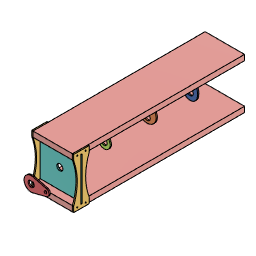
awesomeAutomataCAD (Autodesk Fusion 360 design; units mm, degrees)
Autodesk Fusion 360 part; units mm, degrees
note: some values were not read from the file. Set by a fixed rule: which sketch regions a step uses.
sketch "Sketch1" plane through (0, 0, 0) normal (0, 1, 0) x (1, 0, 0) in component "board"
  line L0 (0, -19.304) -> (139.7, -19.304)
  line L1 (139.7, -19.304) -> (139.7, 0)
  line L2 (139.7, 0) -> (0, 0)
  line L3 (0, 0) -> (0, -19.304)
  dimension "d5" = 139.7
  dimension "d6" = 19.304
  constraint horizontal L0
  constraint vertical L1
  constraint horizontal L2
  constraint vertical L3
  constraint coincident L2.end L3.start
  measures "d5" distance of L0.start L0.end
  measures "d6" distance of L0.start L2.end
extrude "Extrude1" add sketch "Sketch1" along normal blind 609.6 makes body 1 in component "board"
sketch "Sketch2" plane through (139.7, 0, 0) normal (1, 0, 0) x (0, 1, 0) in component "board"
  line L0 (0, 19.304) -> (0, 0)
  line L1 (0, 0) -> (609.6, 0)
  line L2 (609.6, 0) -> (609.6, 19.304)
  line L3 (609.6, 19.304) -> (0, 19.304)
  line L4 (25.4, 19.304) -> (25.4, 12.954)
  line L5 (25.4, 12.954) -> (29.8, 12.954)
  line L6 (29.8, 12.954) -> (29.8, 19.304)
  dimension "d9" = 4.4
  dimension "d10" = 6.35
  dimension "d11" = 25.4
  constraint coincident L3 L4.start
  constraint perpendicular L3 L4
  constraint perpendicular L4 L5
  constraint coincident L3 L6.end
  constraint perpendicular L3 L6
  measures "d9" distance of L4.end L5.end
  measures "d10" distance of L5.end L6.end
  measures "d11" distance of L0.start L4.start
extrude "Extrude2" cut sketch "Sketch2" against normal through all contours L3 L4 L5 L6 bodies 1 in component "board"
copy_body "CopyPasteBodies1" bodies 1 makes body 2 in component "board"
move_body "Move1" bodies 2 to x (1, 0, 0) y (0, -1, 0) z (0, 0, -1) at (0, 0, 0) in component "board"
move_body "Move2" bodies 2 to x (-1, 0, 0) y (0, -1, 0) z (0, 0, 1) at (0, 0, 0) in component "board"
move_body "Move3" bodies 2 to x (1, 0, 0) y (0, 1, 0) z (0, 0, 1) at (139.7, 0, 38.608) in component "board"
move_body "Move4" bodies 2 to x (1, 0, 0) y (0, 1, 0) z (0, 0, 1) at (0, 0, 139.7) in component "board"
sketch "Sketch1 (2)" plane through (0, 0, 0) normal (1, 0, 0) x (0, 1, 0) in component "sideSupport"
  line L0 (29.8, 165.354) -> (29.8, 159.004)
  line L1 (29.8, 159.004) -> (609.6, 159.004)
  line L2 (609.6, 159.004) -> (609.6, 178.308)
  line L3 (609.6, 178.308) -> (0, 178.308)
  line L4 (0, 178.308) -> (0, 159.004)
  line L5 (0, 159.004) -> (25.4, 159.004)
  line L6 (25.4, 159.004) -> (25.4, 165.354)
  line L7 (25.4, 165.354) -> (29.8, 165.354)
  line L8 (29.8, 19.304) -> (29.8, 12.954)
  line L9 (29.8, 12.954) -> (25.4, 12.954)
  line L10 (25.4, 12.954) -> (25.4, 19.304)
  line L11 (25.4, 19.304) -> (0, 19.304)
  line L12 (0, 19.304) -> (0, 0)
  line L13 (0, 0) -> (609.6, 0)
  line L14 (609.6, 0) -> (609.6, 19.304)
  line L15 (609.6, 19.304) -> (29.8, 19.304)
  line L16 (0, 159.004) -> (0, 178.308)
  line L17 (0, 178.308) -> (55.2, 178.308)
  line L18 (55.2, 178.308) -> (55.2, 159.004)
  line L19 (0, 0) -> (55.2, 0)
  line L20 (55.2, 0) -> (55.2, 19.304)
  circle A0 centre (12.7, 168.656) radius 2.032
  circle A1 centre (42.5, 168.656) radius 2.032
  circle A2 centre (12.7, 9.652) radius 2.032
  circle A3 centre (42.5, 9.652) radius 2.032
  line L21 (12.7, 159.004) -> (12.7, 19.304) construction
  line L22 (42.5, 19.304) -> (42.5, 159.004) construction
  spline S0 degree 5 poles (55.2, 19.304) (54.2367, 22.098) (52.3943, 27.686) (49.8831, 36.068) (47.0478, 47.244) (44.4169, 61.214) (42.7808, 75.184) (42.2207, 89.154) (42.7808, 103.124) (44.4169, 117.094) (47.0478, 131.064) (49.8831, 142.24) (52.3943, 150.622) (54.2367, 156.21) (55.2, 159.004) knots 0 0 0 0 0 0 0.1 0.2 0.3 0.4 0.5 0.6 0.7 0.8 0.9 1 1 1 1 1 1
  spline S1 degree 5 poles (0, 159.004) (0.9633, 156.21) (2.8057, 150.622) (5.3169, 142.24) (8.1522, 131.064) (10.7831, 117.094) (12.4192, 103.124) (12.9793, 89.154) (12.4192, 75.184) (10.7831, 61.214) (8.1522, 47.244) (5.3169, 36.068) (2.8057, 27.686) (0.9633, 22.098) (0, 19.304) knots 0 0 0 0 0 0 0.1 0.2 0.3 0.4 0.5 0.6 0.7 0.8 0.9 1 1 1 1 1 1
  line L23 (29.8, 159.004) -> (29.8, 19.304)
  line L24 (25.4, 19.304) -> (25.4, 159.004)
  point P0 (42.5, 89.154)
  point P1 (12.7, 89.154)
  dimension "d18" = 55.2
  dimension "d19" = 55.2
  dimension "d20" = 4.064
  dimension "d21" = 9.652
  dimension "d22" = 12.7
  dimension "d23" = 4.064
  dimension "d24" = 9.652
  dimension "d25" = 12.7
  dimension "d26" = 4.064
  dimension "d27" = 4.064
  dimension "d28" = 9.652
  dimension "d29" = 9.652
  dimension "d30" = 12.7
  dimension "d31" = 12.7
  dimension "d32" = 12.7
  constraint coincident L4.end L5.start
  constraint coincident L3.end L4.start
  constraint perpendicular L16 L17
  constraint coincident L1 L18.end
  constraint perpendicular L1 L18
  constraint coincident L12.end L13.start
  constraint perpendicular L12 L19
  constraint coincident L15 L20.end
  constraint perpendicular L15 L20
  constraint midpoint L5 L21.start
  constraint midpoint L11 L21.end
  constraint coincident L15 L22.start
  constraint coincident L1 L22.end
  constraint perpendicular L1 L22
  constraint midpoint L22 P0
  constraint midpoint L21 P1
  constraint coincident L11.end L12.start
  constraint coincident L0.end L1.start
  constraint coincident L8.start L15.end
  constraint coincident L10.end L11.start
  constraint coincident L5.end L6.start
  measures "d18" distance of L3.end L17.end
  measures "d19" distance of L12.end L19.end
  measures "d20" diameter of A0
  measures "d21" distance of L17 A0.centre
  measures "d22" distance of L16 A0.centre
  measures "d23" diameter of A1
  measures "d24" distance of L17 A1.centre
  measures "d25" distance of L18 A1.centre
  measures "d26" diameter of A2
  measures "d27" diameter of A3
  measures "d28" distance of L11 A2.centre
  measures "d29" distance of L15 A3.centre
  measures "d30" distance of L12 A2.centre
  measures "d31" distance of L20 A3.centre
  measures "d32" distance of L18.end L22
extrude "Extrude1'" add sketch "Sketch1 (2)" against normal blind 4.4 separate body contours L0 L1 L3 L4 L5 L6 L7 L16 L17 L18 | L1 L15 S0 L23 | L8 L9 L10 L11 L12 L13 L15 L19 L20 | L5 L11 S1 L24 makes body 3 in component "sideSupport"
copy_body "CopyPasteBodies1'" bodies 3 makes body 4 in component "sideSupport"
move_body "Move1'" bodies 4 to x (1, 0, 0) y (0, 1, 0) z (0, 0, 1) at (144.1, 0, 0) in component "sideSupport"
sketch "Sketch2 (2)" plane through (0, 29.8, 0) normal (0, -1, 0) x (1, 0, 0) in component "midSupport"
  line L0 (0, 12.954) -> (0, 165.354)
  line L1 (0, 165.354) -> (-4.4, 165.354)
  line L2 (-4.4, 165.354) -> (-4.4, 12.954)
  line L3 (-4.4, 12.954) -> (0, 12.954)
  line L4 (144.1, 12.954) -> (144.1, 165.354)
  line L5 (144.1, 165.354) -> (139.7, 165.354)
  line L6 (139.7, 165.354) -> (139.7, 12.954)
  line L7 (139.7, 12.954) -> (144.1, 12.954)
  line L8 (139.7, 159.004) -> (139.7, 165.354)
  line L9 (139.7, 165.354) -> (0, 165.354)
  line L10 (0, 165.354) -> (0, 159.004)
  line L11 (0, 159.004) -> (139.7, 159.004)
  line L12 (0, 19.304) -> (0, 12.954)
  line L13 (0, 12.954) -> (139.7, 12.954)
  line L14 (139.7, 12.954) -> (139.7, 19.304)
  line L15 (139.7, 19.304) -> (0, 19.304)
  line L16 (144.1, 12.954) -> (-4.4, 165.354) construction
  line L17 (-4.4, 12.954) -> (144.1, 165.354) construction
  circle A0 centre (69.85, 89.154) radius 10.795
  dimension "d35" = 21.59
  constraint coincident L4.start L7.end
  constraint coincident L1.end L2.start
  constraint coincident L2.end L3.start
  constraint coincident L4.end L5.start
  constraint midpoint L17 A0.centre
  measures "d35" diameter of A0
extrude "Extrude1''" add sketch "Sketch2 (2)" along normal blind 4.4 separate body makes body 5 in component "midSupport"
ref_plane "WorkPlane1" through (69.85, 182.2, 89.154) normal (0, 1, 0) x (-1, 0, 0) in component "pearCam"
sketch "Sketch1 (3)" plane through (69.85, 182.2, 95.504) normal (0, 1, 0) x (1, 0, 0) in component "pearCam"
  circle A0 centre (0, 6.35) radius 10.795
  line L0 (74.25, 82.55) -> (-74.25, 82.55)
  line L1 (-74.25, 82.55) -> (-74.25, -69.85)
  line L2 (-74.25, -69.85) -> (74.25, -69.85)
  line L3 (74.25, -69.85) -> (74.25, 82.55)
  circle A1 centre (0, 6.35) radius 21.59
  circle A2 centre (0, -31.75) radius 6.35
  line L4 (19.7876, -2.286) -> (5.8199, -34.29)
  line L5 (-19.7876, -2.286) -> (-5.8199, -34.29)
  line L6 (0, -31.75) -> (0, 6.35) construction
  dimension "d40" = 43.18
  dimension "d41" = 12.7
  dimension "d42" = 38.1
  constraint concentric A0 A1
  constraint coincident A1 L4.start
  constraint coincident A2 L4.end
  constraint tangent A2 L4
  constraint coincident A1 L5.start
  constraint coincident A2 L5.end
  constraint tangent A2 L5
  constraint coincident A2.centre L6.start
  constraint coincident A0.centre A1.centre
  constraint vertical L6
  constraint tangent A1 L5
  constraint tangent A1 L4
  measures "d40" diameter of A1
  measures "d41" diameter of A2
  measures "d42" distance of A0.centre A2.centre
extrude "Extrude1'''" add sketch "Sketch1 (3)" along normal blind 4.4 separate body contours A1 | A1 A2 L4 L5 | A2 makes body 6 in component "pearCam"
ref_plane "WorkPlane1" through (69.85, 334.6, 89.154) normal (0, 1, 0) x (-1, 0, 0) in component "eccentricCam"
sketch "Sketch1 (4)" plane through (69.85, 334.6, 89.154) normal (0, 1, 0) x (1, 0, 0) in component "eccentricCam"
  circle A0 centre (0, 0) radius 10.795
  circle A1 centre (0, -12.7) radius 31.75
  line L0 (0, 0) -> (0, -21.8372) construction
  dimension "d46" = 63.5
  dimension "d47" = 12.7
  constraint coincident A0.centre L0.start
  constraint vertical L0
  constraint coincident A1.centre L0
  measures "d46" diameter of A1
  measures "d47" distance of A0.centre A1.centre
extrude "Extrude1''''" add sketch "Sketch1 (4)" along normal blind 4.4 separate body makes body 7 in component "eccentricCam"
ref_plane "WorkPlane1" through (69.85, 487, 89.154) normal (0, 1, 0) x (-1, 0, 0) in component "snailCam"
sketch "Sketch1 (5)" plane through (69.85, 487, 89.154) normal (0, 1, 0) x (1, 0, 0) in component "snailCam"
  circle A0 centre (0, 0) radius 10.795
  circle A1 centre (0, 0) radius 25.4
  line L0 (0, 0) -> (0, -42.5762)
  arc A2 (7.1494, -46.0115) -> (24.5934, 6.35) centre (-24.5934, -6.35) ccw
  arc A3 (0, -42.5762) -> (7.1494, -46.0115) centre (4.4, -42.5762) ccw
  point P0 (0, -50.8)
  dimension "d51" = 50.8
  dimension "d52" = 50.8
  dimension "d53" = 50.8
  dimension "d54" = 4.4
  constraint concentric A0 A1
  constraint coincident A0.centre A1.centre
  constraint vertical L0
  constraint coincident A1 A2.end
  constraint tangent A1 A2
  constraint coincident P0 L0
  constraint coincident P0 A2
  constraint tangent L0 A3
  constraint tangent A2 A3
  measures "d51" diameter of A1
  measures "d52" distance of A0.centre P0
  measures "d53" radius of A2
  measures "d54" radius of A3
extrude "Extrude1'''''" add sketch "Sketch1 (5)" along normal blind 4.4 separate body makes body 8 in component "snailCam"
ref_plane "WorkPlane1" through (0, -76.2, 0) normal (0, 1, 0) x (0, 0, 1) in component "handle"
sketch "Sketch1 (6)" plane through (0, -76.2, 0) normal (0, 1, 0) x (1, 0, 0) in component "handle"
  circle A0 centre (69.85, -89.154) radius 10.795
  circle A1 centre (69.85, -89.154) radius 25.4
  line L0 (69.85, -89.154) -> (120.65, -89.154) construction
  circle A2 centre (120.65, -89.154) radius 12.7
  circle A3 centre (120.65, -89.154) radius 4.7625
  line L1 (76.2, -64.5606) -> (123.825, -76.8573)
  line L2 (123.825, -101.4507) -> (76.2, -113.7474)
  line L3 (45.8289, -97.409) -> (93.8711, -97.409)
  dimension "d58" = 50.8
  dimension "d59" = 50.8
  dimension "d60" = 25.4
  dimension "d61" = 9.525
  dimension "d62" = 8.255
  constraint concentric A0 A1
  constraint coincident A0.centre A1.centre
  constraint horizontal L0
  constraint coincident L0.end A2.centre
  constraint concentric A2 A3
  constraint coincident A1 L1.start
  constraint coincident A2 L1.end
  constraint coincident A2 L2.start
  constraint coincident A1 L2.end
  constraint tangent A1 L1
  constraint tangent A2 L1
  constraint tangent A2 L2
  constraint tangent A1 L2
  constraint coincident A1 L3.start
  constraint coincident A1 L3.end
  constraint horizontal L3
  measures "d58" diameter of A1
  measures "d59" distance of A0.centre L0.end
  measures "d60" diameter of A2
  measures "d61" diameter of A3
  measures "d62" distance of A0.centre L3
extrude "Extrude1''''''" add sketch "Sketch1 (6)" along normal blind 4.4 separate body contours A0 A1 L3 | A0 L3 | A0 A1 L3 | A1 A2 L1 L2 | A2 picked at (71.7619, -97.7057) makes body 9 in component "handle"
sketch "Sketch1 (7)" plane through (0, -76.2, 0) normal (0, -1, 0) x (1, 0, 0) in component "projectedFront"
  arc A0 (62.8939, 97.409) -> (76.8061, 97.409) centre (69.85, 89.154) ccw
  line L0 (62.8939, 97.409) -> (76.8061, 97.409)
  circle A1 centre (120.65, 89.154) radius 4.7625
  arc A2 (76.2, 113.7474) -> (76.2, 64.5606) centre (69.85, 89.154) ccw
  line L1 (76.2, 64.5606) -> (123.825, 76.8573)
  arc A3 (123.825, 76.8573) -> (123.825, 101.4507) centre (120.65, 89.154) ccw
  line L2 (123.825, 101.4507) -> (76.2, 113.7474)
sketch "Sketch2 (3)" plane through (0, 182.2, 0) normal (0, -1, 0) x (1, 0, 0) in component "projectedFront"
  circle A0 centre (69.85, 89.154) radius 10.795
  arc A1 (50.0624, 97.79) -> (89.6376, 97.79) centre (69.85, 89.154) ccw
  line L0 (89.6376, 97.79) -> (75.6699, 129.794)
  arc A2 (75.6699, 129.794) -> (64.0301, 129.794) centre (69.85, 127.254) ccw
  line L1 (64.0301, 129.794) -> (50.0624, 97.79)
sketch "Sketch3" plane through (0, 334.6, 0) normal (0, -1, 0) x (1, 0, 0) in component "projectedFront"
  circle A0 centre (69.85, 89.154) radius 10.795
  circle A1 centre (69.85, 101.854) radius 31.75
sketch "Sketch4" plane through (0, 487, 0) normal (0, -1, 0) x (1, 0, 0) in component "projectedFront"
  circle A0 centre (69.85, 89.154) radius 10.795
  arc A1 (76.9994, 135.1655) -> (69.85, 131.7302) centre (74.25, 131.7302) ccw
  line L0 (69.85, 131.7302) -> (69.85, 114.554)
  arc A2 (69.85, 114.554) -> (94.4434, 82.804) centre (69.85, 89.154) ccw
  arc A3 (94.4434, 82.804) -> (76.9994, 135.1655) centre (45.2566, 95.504) ccw
sketch "Sketch5" plane through (0, 25.4, 0) normal (0, -1, 0) x (1, 0, 0) in component "projectedFront"
  circle A0 centre (69.85, 89.154) radius 10.795
  line L0 (-4.4, 12.954) -> (144.1, 12.954)
  line L1 (144.1, 12.954) -> (144.1, 165.354)
  line L2 (144.1, 165.354) -> (-4.4, 165.354)
  line L3 (-4.4, 165.354) -> (-4.4, 12.954)
sketch "Sketch1 (8)" plane through (144.1, 0, 0) normal (1, 0, 0) x (0, 1, 0) in component "projectedSide"
  line L0 (25.4, 12.954) -> (25.4, 165.354)
  line L1 (25.4, 165.354) -> (29.8, 165.354)
  line L2 (29.8, 165.354) -> (29.8, 12.954)
  line L3 (29.8, 12.954) -> (25.4, 12.954)
  circle A0 centre (42.5, 9.652) radius 2.032
  circle A1 centre (12.7, 9.652) radius 2.032
  circle A2 centre (42.5, 168.656) radius 2.032
  circle A3 centre (12.7, 168.656) radius 2.032
  line L4 (0, 178.308) -> (0, 159.004)
  spline S0 degree 5 poles (0, 159.004) (0.9633, 156.21) (2.8057, 150.622) (5.3169, 142.24) (8.1522, 131.064) (10.7831, 117.094) (12.4192, 103.124) (12.9793, 89.154) (12.4192, 75.184) (10.7831, 61.214) (8.1522, 47.244) (5.3169, 36.068) (2.8057, 27.686) (0.9633, 22.098) (0, 19.304) knots 0 0 0 0 0 0 0.1 0.2 0.3 0.4 0.5 0.6 0.7 0.8 0.9 1 1 1 1 1 1
  line L5 (0, 19.304) -> (0, 0)
  line L6 (0, 0) -> (55.2, 0)
  line L7 (55.2, 0) -> (55.2, 19.304)
  spline S1 degree 5 poles (55.2, 19.304) (54.2367, 22.098) (52.3943, 27.686) (49.8831, 36.068) (47.0478, 47.244) (44.4169, 61.214) (42.7808, 75.184) (42.2207, 89.154) (42.7808, 103.124) (44.4169, 117.094) (47.0478, 131.064) (49.8831, 142.24) (52.3943, 150.622) (54.2367, 156.21) (55.2, 159.004) knots 0 0 0 0 0 0 0.1 0.2 0.3 0.4 0.5 0.6 0.7 0.8 0.9 1 1 1 1 1 1
  line L8 (55.2, 159.004) -> (55.2, 178.308)
  line L9 (55.2, 178.308) -> (0, 178.308)
component "board" placed x (1, 0, 0) y (0, 1, 0) z (0, 0, 1) at (0, 0, 0)
component "sideSupport" placed x (1, 0, 0) y (0, 1, 0) z (0, 0, 1) at (0, 0, 0)
component "midSupport" placed x (1, 0, 0) y (0, 1, 0) z (0, 0, 1) at (0, 0, 0)
component "pearCam" placed x (1, 0, 0) y (0, 1, 0) z (0, 0, 1) at (0, 0, 0)
component "eccentricCam" placed x (1, 0, 0) y (0, 1, 0) z (0, 0, 1) at (0, 0, 0)
component "snailCam" placed x (1, 0, 0) y (0, 1, 0) z (0, 0, 1) at (0, 0, 0)
component "handle" placed x (1, 0, 0) y (0, 1, 0) z (0, 0, 1) at (0, 0, 0)
component "projectedSide" placed x (1, 0, 0) y (0, 1, 0) z (0, 0, 1) at (0, 0, 0)
component "projectedFront" placed x (1, 0, 0) y (0, 1, 0) z (0, 0, 1) at (0, 0, 0)
equation "boardW = 5.5 in"
equation "boardThick = 0.76 in"
equation "boardL = 2 ft"
equation "plyThick = 4.4 mm"
equation "d5 = boardW"
equation "d6 = boardThick"
equation "d7 = boardL"
equation "d9 = plyThick"
equation "d18 = 2 in + plyThick"
equation "d19 = 2 in + plyThick"
equation "d21 = boardThick / 2"
equation "d24 = boardThick / 2"
equation "d28 = boardThick / 2"
equation "d29 = boardThick / 2"
equation "d33 = -plyThick"
equation "d35 = poleD"
equation "d36 = plyThick"
equation "poleD = 0.85 in"
equation "d40 = poleD * 2"
equation "d43 = plyThick"
equation "d48 = plyThick"
equation "d54 = plyThick"
equation "d55 = plyThick"
equation "d62 = poleD / 2 - 0.1 in"
equation "d63 = plyThick"
